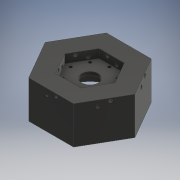
# Autodesk Inventor part: XT-SM-04
Saved by Autodesk Inventor 2017 (Build 210142000, 142)
## iProperties
Created: 2019-11-11
Part Number: XT-SM-04
Material: ABS Plastic
Document SubType Name: Modeling
Designer: Dell
Density: 1.06 g/cm^3
Appearance: Smooth - Black
Author: Dell
Autodesk Inventor part; units mm, degrees
ref_plane "YZ Plane" through (0, 0, 0) normal (1, 0, 0) x (0, 1, 0)
ref_plane "XZ Plane" through (0, 0, 0) normal (0, 1, 0) x (-1, 0, 0)
ref_plane "XY Plane" through (0, 0, 0) normal (0, 0, 1) x (1, 0, 0)
sketch "Sketch1" plane through (0, 0, 0) normal (0, 0, 1) x (1, 0, 0)
  line L0 (68.1273, 0) -> (34.0637, -59)
  line L1 (34.0637, -59) -> (-34.0637, -59)
  line L2 (-34.0637, -59) -> (-68.1273, 0)
  line L3 (-68.1273, 0) -> (-34.0637, 59)
  line L4 (-34.0637, 59) -> (34.0637, 59)
  line L5 (34.0637, 59) -> (68.1273, 0)
  circle A0 centre (0, 0) radius 56
  dimension "d0" = 118
  dimension "d2" = 112
  constraints: 12 end point, 2 coincident, 1 centre point, 1 horizontal, 13 other
  measures "d0" distance between parallel lines of L1 L4
  measures "d2" diameter of A0
extrude "Extrusion1" add sketch "Sketch1" along normal blind 39
sketch "Sketch3" plane through (0, 0, 39) normal (0, 0, 1) x (1, 0, 0)
  circle A0 centre (0, 0) radius 12.5
  line L0 (-34.0637, 59) -> (-68.1273, 0) projected
  line L1 (-68.1273, 0) -> (-34.0637, 59)
  line L2 (-34.0637, 59) -> (34.0637, 59)
  line L3 (34.0637, 59) -> (68.1273, 0)
  line L4 (68.1273, 0) -> (34.0637, -59)
  line L5 (34.0637, -59) -> (-34.0637, -59)
  line L6 (-34.0637, -59) -> (-68.1273, 0)
  circle A1 centre (29.5, 0) radius 2.25
  circle A2 centre (20.8597, 20.8597) radius 2.25
  circle A3 centre (0, 29.5) radius 2.25
  circle A4 centre (-20.8597, 20.8597) radius 2.25
  circle A5 centre (-29.5, 0) radius 2.25
  circle A6 centre (-20.8597, -20.8597) radius 2.25
  circle A7 centre (0, -29.5) radius 2.25
  circle A8 centre (20.8597, -20.8597) radius 2.25
  dimension "d5" = 25
  dimension "d8" = 29.5
  dimension "d9" = 4.5
  dimension "d12" = 360
  constraints: 12 end point, 9 centre point, 2 coincident, 1 horizontal alignment, 30 other
  measures "d5" diameter of A0
  measures "d8" distance of A1.centre point (0, 0)
  measures "d9" diameter of A1
extrude "Extrusion2" add sketch "Sketch3" along normal blind 5
sketch "Sketch4" plane through (0, 0, 44) normal (0, 0, 1) x (1, 0, 0)
  line L0 (-38.1051, 0) -> (-19.0526, 33)
  line L1 (-19.0526, 33) -> (19.0526, 33)
  line L2 (19.0526, 33) -> (38.1051, 0)
  line L3 (38.1051, 0) -> (19.0526, -33)
  line L4 (19.0526, -33) -> (-19.0526, -33)
  line L5 (-19.0526, -33) -> (-38.1051, 0)
  line L6 (-68.1273, 0) -> (-34.0637, 59)
  line L7 (-34.0637, 59) -> (34.0637, 59)
  line L8 (34.0637, 59) -> (68.1273, 0)
  line L9 (68.1273, 0) -> (34.0637, -59)
  line L10 (34.0637, -59) -> (-34.0637, -59)
  line L11 (-34.0637, -59) -> (-68.1273, 0)
  point P0 (0, 0)
  point P1 (0, 0)
  point P2 (0, 0)
  dimension "d14" = 66
  constraints: 24 end point, 3 coincident, 1 horizontal, 26 other
  measures "d14" distance between parallel lines of L4 L1
extrude "Extrusion3" add sketch "Sketch4" along normal blind 13
sketch "Sketch5" plane through (-34.0637, 59, 0) normal (0, 1, 0) x (1, 0, 0)
  line L0 (53.1162, -44) -> (15.0111, -44) projected
  line L1 (53.1162, -44) -> (53.1162, -57) projected
  line L2 (15.0111, -57) -> (53.1162, -57) projected
  line L3 (15.0111, -44) -> (15.0111, -57) projected
  line L4 (26.9926, -53) -> (41.1347, -48)
  circle A0 centre (26.9926, -53) radius 2.5
  circle A1 centre (41.1347, -48) radius 2.5
  point P0 (34.0637, 0)
  point P1 (34.0637, -50.5)
  point P2 (34.0637, -57)
  point P3 (15.0111, -50.5)
  dimension "d17" = 5
  dimension "d18" = 5
  dimension "d19" = 15
  dimension "d20" = 5
  constraints: 3 midpoint, 2 centre point, 2 coincident, 2 end point, 1 horizontal alignment, 1 vertical alignment
  measures "d17" diameter of A0
  measures "d18" diameter of A1
  measures "d19" distance of L4.start L4.end
  measures "d20" vertical distance of A0.centre A1.centre
extrude "Extrusion4" cut sketch "Sketch5" against normal up to surface (26 mm away) from surface at 0 contours A0 | A1
pattern_circular "Circular Pattern1" count 6 over 360 about axis through (0, 0, 39) along (0, 0, 1) of "Extrusion4"
body "Solid1"
